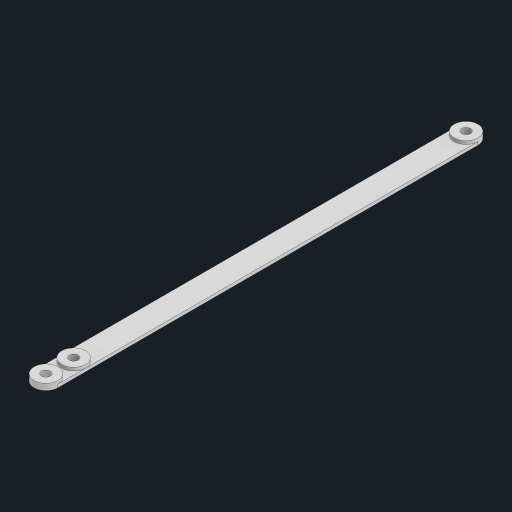
# Autodesk Inventor part: közepső szalag 1
Saved by Autodesk Inventor 2023 (Build 270158000, 158)
## iProperties
Created: 2022-11-11
Part Number: közepső szalag 1
Material: Generic
Document SubType Name: Modeling
Designer: gd1
Density: 1 g/cm^3
Appearance: Default
Mass: 4.85227 g
Surface Area: 91.2689 cm^2
Volume: 4.85227 cm^3
Author: gd1
Autodesk Inventor part; units mm, degrees
ref_plane "YZ Plane" through (0, 0, 0) normal (1, 0, 0) x (0, 1, 0)
ref_plane "XZ Plane" through (0, 0, 0) normal (0, 1, 0) x (-1, 0, 0)
ref_plane "XY Plane" through (0, 0, 0) normal (0, 0, 1) x (1, 0, 0)
sketch "Sketch1" plane through (0, 0, 0) normal (0, 1, 0) x (-1, 0, 0)
  circle A0 centre (0, 0) radius 7.5
  circle A1 centre (0, 0) radius 2.75
  line L0 (-7.5, -247.97) -> (-7.5, 0)
  line L1 (7.5, 0) -> (7.5, -247.97)
  arc A2 (7.5, 0) -> (-7.5, 0) centre (0, 0) ccw
  line L2 (0, -255.47) -> (0, -240.47)
  circle A3 centre (0, -247.97) radius 2.75
  circle A4 centre (0, -247.97) radius 7.5
  line L3 (-7.5, 7.5) -> (-7.5, 10)
  line L4 (7.5, 10) -> (7.5, 7.5)
  line L5 (-7.5, 10) -> (-7.5, 17.5)
  line L6 (7.5, 17.5) -> (7.5, 10)
  circle A5 centre (0, 17.5) radius 7.5
  circle A6 centre (0, 17.5) radius 2.75
  line L7 (7.5, 7.5) -> (7.5, 0)
  line L8 (-7.5, 7.5) -> (-7.5, 0)
  line L9 (7.5, 0) -> (7.5, -247.97)
  line L10 (7.5, -123.985) -> (-7.5, -123.985)
  line L11 (-7.5, -255.47) -> (-7.5, -257.97)
  line L12 (7.5, -257.97) -> (7.5, -255.47)
  line L13 (-7.5, -257.97) -> (-7.5, -265.47)
  line L14 (7.5, -265.47) -> (7.5, -257.97)
  circle A7 centre (0, -265.47) radius 7.5
  circle A8 centre (0, -265.47) radius 2.75
  line L15 (7.5, -255.47) -> (7.5, -247.97)
  line L16 (-7.5, -255.47) -> (-7.5, -247.97)
  point P0 (7.5, 0)
  point P1 (-7.5, 0)
  point P2 (0, 7.5)
  point P3 (7.5, 0)
  dimension "d0" = 15
  dimension "d1" = 5.5
  dimension "d7" = 15
  dimension "d12" = 15
  dimension "d13" = 5.5
  dimension "d17" = 262.97
  dimension "d18" = 15
  dimension "d19" = 2.5
  dimension "d22" = 15
  dimension "d23" = 5.5
  constraints: 34 end point, 10 point on circle, 10 symmetric about line, 8 centre point, 5 coincident, 3 midpoint, 3 parallel, 3 tangent, 1 point on line, 1 vertical, 5 other
  measures "d1" diameter of A1
  measures "d7" distance between parallel lines of L0 L1
  measures "d12" distance of L2.start L2.end
  measures "d13" diameter of A3
  measures "d17" distance of point (0, 7.5) L2.start
  measures "d18" distance of L3.end L4.start
  measures "d19" distance of L3.start L3.end
  measures "d22" diameter of A5
  measures "d23" diameter of A6
extrude "Extrusion2" add sketch "Sketch1" along normal blind 4 contours A0 | A4 L2 A3 | A4 L2 A3 | A5
extrude "Extrusion3" add sketch "Sketch1" along normal blind 2 contours L1 L10 L0 A0 | A0 L8 L3 L5 A5 L6 L4 L7 | L1 A4 L0 L10 | A5
body "Solid1"
